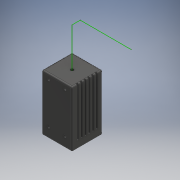
# Autodesk Inventor part: Laser
Saved by Autodesk Inventor 2017 (Build 210142000, 142)
## iProperties
Part Number: Laser
Material: Aluminium 6061
Document SubType Name: Modeling
Designer: Adrien MARY
Density: 2.7 g/cm^3
Appearance: Aluminium - Plat(1)
Mass: 127.285 g
Surface Area: 111.688 cm^2
Volume: 47.1425 cm^3
Stock Number: 1410-03-09
Project: 1410 LaserShow
Author: Adrien MARY
Autodesk Inventor part; units mm, degrees
ref_plane "YZ Plane" through (0, 0, 0) normal (1, 0, 0) x (0, 1, 0)
ref_plane "XZ Plane" through (0, 0, 0) normal (0, 1, 0) x (-1, 0, 0)
ref_plane "XY Plane" through (0, 0, 0) normal (0, 0, 1) x (1, 0, 0)
sketch "Esquisse1" plane through (0, 0, 0) normal (0, 0, 1) x (1, 0, 0)
  line L0 (-15, -15) -> (15, -15)
  line L1 (15, -15) -> (15, 15)
  line L2 (15, 15) -> (-15, 15)
  line L3 (-15, 15) -> (-15, -15)
  line L4 (-15, -15) -> (15, 15) construction
  line L5 (15, -15) -> (-15, 15) construction
  point P0 (0, 0)
  dimension "d0" = 30
  dimension "d1" = 30
  constraints: 12 end point, 2 midpoint, 2 parallel, 1 horizontal, 1 perpendicular
  measures "d0" distance of L2.end L1.end
  measures "d1" distance of L1.end L0.end
extrude "Extrusion1" add sketch "Esquisse1" along normal mid plane 55
sketch "Esquisse2" plane through (-15, -15, 27.5) normal (0, -1, 0) x (1, 0, 0)
  line L0 (0, 0) -> (30, 0) projected
  point P0 (15, -27.5)
  point P1 (7, -5)
  point P2 (23, -5)
  point P3 (23, -45)
  point P4 (7, -45)
  dimension "d4" = 40
  dimension "d5" = 16
  dimension "d6" = 8
  dimension "d7" = 5
  constraints: 2 horizontal alignment, 2 vertical alignment
  measures "d4" distance of point (23, -5) point (23, -45)
  measures "d5" distance of point (7, -5) point (23, -5)
  measures "d6" horizontal distance of point (23, -5) point (15, -27.5)
  measures "d7" distance from line of L0 point (23, -5)
hole "Perçage1" at (-8, -15, 22.5) at (8, -15, 22.5) at (8, -15, -17.5) at (-8, -15, -17.5) direction (0, 1, 0) diameter 2.459 depth 8.8 tip angle 118 thread size "M3x0.5" class "6H" standard "ISO Metric profile"
sketch "Esquisse3" plane through (0, 0, 27.5) normal (0, 0, 1) x (1, 0, 0)
  circle A0 centre (0, 0) radius 1.5
  dimension "d15" = 3
  constraints: 1 centre point, 1 coincident
  measures "d15" diameter of A0
extrude "Extrusion2" cut sketch "Esquisse3" against normal blind 10
sketch "Esquisse4" plane through (0, 0, 17.5) normal (0, 0, 1) x (1, 0, 0)
  circle A0 centre (0, 0) radius 0.2
  dimension "d19" = 0.4
  constraints: 1 centre point, 1 coincident
  measures "d19" diameter of A0
extrude "Extrusion3" [suppressed]
sketch "Esquisse5" plane through (0, 0, 27.5) normal (0, 0, 1) x (1, 0, 0)
  line L0 (-20, -10) -> (-13.5, -10)
  line L1 (-13.5, -10) -> (-13.5, -8.5)
  line L2 (-13.5, -8.5) -> (-20, -8.5)
  line L3 (-20, -8.5) -> (-20, -10)
  line L4 (-15, -15) -> (15, -15) projected
  line L5 (-15, 15) -> (-15, -15) projected
  line L6 (15, 15) -> (-15, 15) projected
  line L7 (-20, -6.3) -> (-13.5, -6.3)
  line L8 (-13.5, -6.3) -> (-13.5, -4.8)
  line L9 (-13.5, -4.8) -> (-20, -4.8)
  line L10 (-20, -4.8) -> (-20, -6.3)
  line L11 (-20, -2.6) -> (-13.5, -2.6)
  line L12 (-13.5, -2.6) -> (-13.5, -1.1)
  line L13 (-13.5, -1.1) -> (-20, -1.1)
  line L14 (-20, -1.1) -> (-20, -2.6)
  line L15 (-20, 1.1) -> (-13.5, 1.1)
  line L16 (-13.5, 1.1) -> (-13.5, 2.6)
  line L17 (-13.5, 2.6) -> (-20, 2.6)
  line L18 (-20, 2.6) -> (-20, 1.1)
  line L19 (-20, 4.8) -> (-13.5, 4.8)
  line L20 (-13.5, 4.8) -> (-13.5, 6.3)
  line L21 (-13.5, 6.3) -> (-20, 6.3)
  line L22 (-20, 6.3) -> (-20, 4.8)
  line L23 (-20, 8.5) -> (-13.5, 8.5)
  line L24 (-13.5, 8.5) -> (-13.5, 10)
  line L25 (-13.5, 10) -> (-20, 10)
  line L26 (-20, 10) -> (-20, 8.5)
  point P0 (0, 0)
  dimension "d22" = 5
  dimension "d23" = 1.5
  dimension "d24" = 1.5
  dimension "d25" = 30
  dimension "d26" = 5
  dimension "d29" = 3.7
  dimension "d34" = 5
  constraints: 48 end point, 2 parallel, 1 horizontal, 1 perpendicular, 1 vertical, 40 other
  measures "d22" distance between parallel lines of L4 L0
  measures "d23" distance between parallel lines of L2 L0
  measures "d24" distance between parallel lines of L5 L1
  measures "d25" distance between parallel lines of L6 L4
  measures "d26" distance between parallel lines of L5 L3
  measures "d29" distance of L0.start L7.start
  measures "d34" distance between parallel lines of L6 L25
extrude "Extrusion4" cut sketch "Esquisse5" against normal blind 47.5
pattern_circular "Réseau circulaire1" count 2 over 90 about axis through (0, 0, -10) along (0, 0, -1) of "Extrusion4"
mirror "Symétrie1" about plane through (0, 0, 0) normal (1, 0, 0) of "Extrusion4"
fillet "Congé1" radius 1.5 30 edges at (15, 15, 0) (15, -15, 0) (-15, -15, 0) (-15, 12.5, 27.5) (-15, 7.4, 27.5) (-15, 0, 27.5) (-15, -7.4, 27.5) (-15, -12.5, 27.5) (-15, -3.7, 27.5) (-15, 3.7, 27.5) (0, -15, 27.5) (15, -12.5, 27.5) (15, 12.5, 27.5) (15, 3.7, 27.5) (15, -3.7, 27.5) (15, -7.4, 27.5) (15, 0, 27.5) (15, 7.4, 27.5) (12.5, 15, 27.5) (7.4, 15, 27.5) (0, 15, 27.5) (-7.4, 15, 27.5) (-12.5, 15, 27.5) (-3.7, 15, 27.5) (3.7, 15, 27.5) (15, 0, -27.5) (0, 15, -27.5) (-15, 0, -27.5) (0, -15, -27.5) (-15, 15, 0)
sketch "Esquisse9" plane through (0, 0, 17.5) normal (0, 0, 1) x (1, 0, 0)
  circle A0 centre (0, 0) radius 0.2
  dimension "d50" = 0.4
  constraints: 1 centre point, 1 coincident
  measures "d50" diameter of A0
extrude "Extrusion8" add sketch "Esquisse9" along normal blind 48
sketch "Esquisse6" plane through (0, 0, 0) normal (0, 1, 0) x (-1, 0, 0)
  circle A0 centre (0, 65.5) radius 0.2
  line L0 (0.2, 65.5) -> (-0.2, 65.5) construction
  point P0 (0, 0)
  dimension "d40" = 0.4
  constraints: 1 centre point, 1 coincident, 1 midpoint
  measures "d40" diameter of A0
extrude "Extrusion5" add sketch "Esquisse6" along normal blind 8
sketch "Esquisse7" plane through (0, 0, 0) normal (1, 0, 0) x (0, 1, 0)
  line L0 (8, 65.3) -> (8, 65.7) projected
  circle A0 centre (8, 65.5) radius 0.2
  point P0 (0, 0)
  dimension "d44" = 0.4
  constraints: 1 centre point, 1 midpoint
  measures "d44" diameter of A0
extrude "Extrusion6" add sketch "Esquisse7" along normal blind 50
sketch "Esquisse11" plane through (-15, -13.5, -26) normal (-1, 0, 0) x (0, 0, 1)
  line L0 (0, -1.5) -> (52, -1.5) projected
  line L1 (-1.5, 27) -> (-1.5, 0) projected
  point P0 (26, 13.5)
  point P1 (1.5, 1.5)
  point P2 (3.5, 1.5)
  point P3 (5.5, 1.5)
  point P4 (7.5, 1.5)
  point P5 (9.5, 1.5)
  dimension "d56" = 2
  dimension "d57" = 2
  dimension "d58" = 2
  dimension "d59" = 2
  dimension "d60" = 3
  dimension "d61" = 3
  constraints: 4 horizontal alignment
  measures "d56" distance of point (1.5, 1.5) point (3.5, 1.5)
  measures "d57" distance of point (5.5, 1.5) point (3.5, 1.5)
  measures "d58" distance of point (5.5, 1.5) point (7.5, 1.5)
  measures "d59" distance of point (7.5, 1.5) point (9.5, 1.5)
  measures "d60" distance from line of L0 point (1.5, 1.5)
  measures "d61" distance from line of L1 point (1.5, 1.5)
sketch "Esquisse12" plane through (0, 0, -27.5) normal (0, 0, -1) x (-1, 0, 0)
  point P0 (0, 0)
  point P1 (-12, -12)
  point P2 (-12, 12)
  point P3 (12, 12)
  point P4 (12, -12)
  dimension "d62" = 24
  dimension "d63" = 12
  dimension "d64" = 24
  dimension "d65" = 12
  constraints: 2 horizontal alignment, 2 vertical alignment
  measures "d62" distance of point (12, 12) point (-12, 12)
  measures "d63" horizontal distance of point (0, 0) point (12, 12)
  measures "d64" distance of point (12, 12) point (12, -12)
  measures "d65" horizontal distance of point (0, 0) point (12, 12)
hole "Perçage2" at (12, -12, -27.5) at (12, 12, -27.5) at (-12, 12, -27.5) at (-12, -12, -27.5) direction (0, 0, 1) diameter 2.459 depth 8.8 tip angle 118 thread size "M3x0.5" class "6H" standard "ISO Metric profile"
equation "\"d6\" = 0.5 * d5"
equation "\"d24\" = d23"
equation "\"d57\" = d56"
equation "\"d58\" = d57"
equation "\"d59\" = d58"
equation "\"d61\" = d60"
equation "\"d63\" = 0.5 * d64"
equation "\"d64\" = d62"
equation "\"d65\" = 0.5 * d62"
equation "\"pi\" = 3.141593"
equation "\"nombredor\" = 1.61803"
